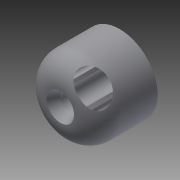
# Autodesk Inventor part: adaptor
Saved by Autodesk Inventor 2015 (Build 190159000, 159)
## iProperties
Created: 2014-10-25
Part Number: adaptor
Material: Generic
Document SubType Name: Modeling
Designer: jesse
Density: 1 g/cm^3
Appearance: Default
Author: jesse
Autodesk Inventor part; units mm, degrees
ref_plane "YZ Plane" through (0, 0, 0) normal (1, 0, 0) x (0, 1, 0)
ref_plane "XZ Plane" through (0, 0, 0) normal (0, 1, 0) x (-1, 0, 0)
ref_plane "XY Plane" through (0, 0, 0) normal (0, 0, 1) x (1, 0, 0)
sketch "Sketch1" plane through (0, 0, 0) normal (0, 0, 1) x (1, 0, 0)
  circle A0 centre (0, 0) radius 13.2282
  circle A1 centre (0, 0) radius 3.05
  circle A2 centre (-8, 0) radius 1.3525
  circle A3 centre (0, 8) radius 1.3525
  circle A4 centre (8, 0) radius 1.3525
  circle A5 centre (0, -8) radius 1.3525
  dimension "d12" = 6.1
  dimension "d13" = 2.705
  dimension "d14" = 2.705
  dimension "d15" = 2.705
  dimension "d16" = 2.705
  constraints: 6 centre point
  measures "d12" diameter of A1
  measures "d13" diameter of A2
  measures "d14" diameter of A5
  measures "d15" diameter of A4
  measures "d16" diameter of A3
extrude "Extrusion1" add sketch "Sketch1" along normal blind 12.7
sketch "Sketch7" plane through (0, 0, 12.7) normal (0, 0, 1) x (1, 0, 0)
  circle A0 centre (0, 0) radius 3.05
  circle A1 centre (0, 0) radius 13.2282 projected
  constraints: 1 centre point, 1 coincident
extrude "Extrusion6" add sketch "Sketch7" along normal blind 7.9375
fillet "Fillet2" radius 7.9375 1 edges at (-13.2282, 0, 20.6375)
sketch "Sketch8" plane through (0, 0, 0) normal (0, 0, -1) x (-1, 0, 0)
  circle A0 centre (0, 0) radius 3.175
  dimension "d21" = 6.35
  constraints: 1 centre point, 1 coincident
  measures "d21" diameter of A0
extrude "Extrusion7" cut sketch "Sketch8" against normal through all
chamfer "Chamfer1" distance 1.5875 distance2 3.175 1 edges at (3.175, 0, 20.6375) measured on face at (4.5034, -0.6753, 20.6375)
body "Solid1"
